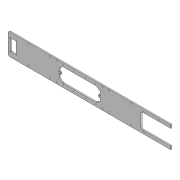
# Autodesk Inventor part: SlipersLåda 211018006
Saved by Autodesk Inventor 2020 (Build 240168000, 168)
## iProperties
Created: 2021-10-19
Part Number: SlipersLåda 211018006
Material: Generic
Document SubType Name: Modeling
Designer: dicpet001
Density: 1 g/cm^3
Appearance: Default
Author: dicpet001
Autodesk Inventor part; units mm, degrees
ref_plane "YZ Plane" through (0, 0, 0) normal (1, 0, 0) x (0, 1, 0)
ref_plane "XZ Plane" through (0, 0, 0) normal (0, 1, 0) x (-1, 0, 0)
ref_plane "XY Plane" through (0, 0, 0) normal (0, 0, 1) x (1, 0, 0)
sketch "Sketch1" plane through (0, 0, 0) normal (0, 0, 1) x (1, 0, 0)
  line L0 (0, 288.6985) -> (0, -288.6985) projected
  line L1 (-2107.4558, 0) -> (2101.2426, 0) projected
  line L2 (-1470, 200) -> (1500, 200)
  line L3 (1500, 200) -> (1500, -200)
  line L4 (1500, -200) -> (-1470, -200)
  line L5 (-1500, -170) -> (-1500, 170)
  arc A0 (-1470, 200) -> (-1500, 170) centre (-1470, 170) ccw
  arc A1 (-1500, -170) -> (-1470, -200) centre (-1470, -170) ccw
  line L6 (-1445, 110) -> (-1365, 110)
  line L7 (-1350, 95) -> (-1350, -95)
  line L8 (-1365, -110) -> (-1445, -110)
  line L9 (-1460, -95) -> (-1460, 95)
  arc A2 (-1445, 110) -> (-1460, 95) centre (-1445, 95) ccw
  arc A3 (-1350, 95) -> (-1365, 110) centre (-1365, 95) ccw
  arc A4 (-1365, -110) -> (-1350, -95) centre (-1365, -95) ccw
  arc A5 (-1460, -95) -> (-1445, -110) centre (-1445, -95) ccw
  point P0 (0, 0)
  point P1 (-1500, 200)
  point P2 (-1500, -200)
  point P3 (-1465, 115)
  point P4 (-1345, 115)
  point P5 (-1345, -115)
  point P6 (-1465, -115)
  dimension "d0" = 400
  dimension "d1" = 3000
  dimension "d2" = 30
  dimension "d3" = 110
  dimension "d4" = 220
  dimension "d5" = 15
  dimension "d8" = 230
  dimension "d9" = 120
  dimension "d10" = 5
  dimension "d11" = 5
  dimension "d12" = 40
  constraints: 16 end point, 12 point on circle, 12 tangent, 6 centre point, 4 equal radius, 4 parallel, 4 point on line, 2 horizontal, 2 horizontal alignment, 2 perpendicular, 2 vertical alignment, 3 other
  measures "d0" distance of point (-1500, -200) point (-1500, 200)
  measures "d1" distance of point (-1500, 200) L2.end
  measures "d2" radius of A0
  measures "d3" distance between parallel lines of L7 L9
  measures "d4" distance between parallel lines of L8 L6
  measures "d5" radius of A2
  measures "d8" distance of point (-1345, -115) point (-1345, 115)
  measures "d9" distance of point (-1465, -115) point (-1345, -115)
  measures "d10" distance from line of L8 point (-1465, -115)
  measures "d11" distance from line of L9 point (-1465, -115)
  measures "d12" distance between parallel lines of L9 L5
extrude "Extrusion1" add sketch "Sketch1" against normal blind 20 contours L2 L3 L1 L0 | L0 L1 L7 A3 L6 A2 L9 L5 A0 L2 | L1 L3 L4 L0 | L0 L4 A1 L5 L1 L9 A5 L8 A4 L7
hole "Hole1" at (-1465, 115, 0) at (-1345, 115, 0) at (-1345, -115, 0) at (-1465, -115, 0) direction (0, 0, -1) diameter 10.106 end through all thread size "M12x1.75" class "6H" standard "ISO Metric profile"
sketch "Sketch2" plane through (0, 0, 0) normal (0, 0, 1) x (1, 0, 0)
  circle A0 centre (-1345, -115) radius 5.053 projected
  circle A1 centre (-1465, 115) radius 5.053 projected
  circle A2 centre (-1345, 115) radius 5.053 projected
  circle A3 centre (-1465, -115) radius 5.053 projected
  line L0 (-1500, 170) -> (-1500, -170) projected
  arc A4 (-1500, -170) -> (-1470, -200) centre (-1470, -170) ccw projected
  line L1 (-1470, -200) -> (1500, -200) projected
  line L2 (1500, -200) -> (1500, 200) projected
  line L3 (1500, 200) -> (-1470, 200) projected
  arc A5 (-1470, 200) -> (-1500, 170) centre (-1470, 170) ccw projected
  arc A6 (-1460, -95) -> (-1445, -110) centre (-1445, -95) ccw projected
  line L4 (-1460, -95) -> (-1460, 95) projected
  arc A7 (-1445, 110) -> (-1460, 95) centre (-1445, 95) ccw projected
  line L5 (-1445, 110) -> (-1365, 110) projected
  arc A8 (-1350, 95) -> (-1365, 110) centre (-1365, 95) ccw projected
  line L6 (-1350, 95) -> (-1350, -95) projected
  arc A9 (-1365, -110) -> (-1350, -95) centre (-1365, -95) ccw projected
  line L7 (-1365, -110) -> (-1445, -110) projected
  line L8 (1500, 140) -> (975, 140)
  line L9 (950, 115) -> (950, -115)
  line L10 (975, -140) -> (1500, -140)
  line L11 (1500, -140) -> (1500, 140)
  line L12 (0, 288.6985) -> (0, -288.6985) projected
  line L13 (-2107.4558, 0) -> (2101.2426, 0) projected
  arc A10 (975, 140) -> (950, 115) centre (975, 115) ccw
  arc A11 (950, -115) -> (975, -140) centre (975, -115) ccw
  circle A12 centre (1270, 175) radius 3.5
  point P0 (0, 0)
  point P1 (998, 160)
  point P2 (1025, 160)
  point P3 (998, -160)
  point P4 (1025, -160)
  point P5 (1270, 160)
  dimension "d22" = 550
  dimension "d23" = 280
  dimension "d24" = 25
  dimension "d25" = 7
  dimension "d26" = 230
  dimension "d27" = 320
  dimension "d28" = 27
  dimension "d29" = 475
  dimension "d30" = 230
  dimension "d31" = 15
  constraints: 8 end point, 4 point on circle, 4 tangent, 3 centre point, 3 horizontal alignment, 2 parallel, 2 vertical alignment, 1 equal radius, 1 horizontal, 1 perpendicular, 1 point on line, 1 symmetric about line, 1 other
  measures "d22" distance between parallel lines of L2 L9
  measures "d23" distance between parallel lines of L10 L8
  measures "d24" radius of A10
  measures "d25" diameter of A12
  measures "d26" distance from line of L2 A12.centre
  measures "d27" distance of point (1025, -160) point (1025, 160)
  measures "d28" distance of point (998, 160) point (1025, 160)
  measures "d29" distance from line of L2 point (1025, -160)
  measures "d30" distance from line of L2 point (1270, 160)
  measures "d31" distance of A12.centre point (1270, 160)
extrude "Extrusion2" cut sketch "Sketch2" against normal blind 20 contours L2 L13 L9 A10 L8 | L13 L2 L10 A11 L9 | A12
hole "Hole2" at (998, 160, 0) at (1025, 160, 0) at (998, -160, 0) at (1025, -160, 0) at (1270, 160, 0) direction (0, 0, -1) diameter 10.106 end through all thread size "M12x1.75" class "6H" standard "ISO Metric profile"
sketch "Sketch3" plane through (0, 0, 0) normal (0, 0, 1) x (1, 0, 0)
  line L0 (0, 1076.2642) -> (0, -784.2642) projected
  line L1 (-2100, 0) -> (2100, 0) projected
  line L2 (1500, -200) -> (1500, -140) projected
  line L3 (-1470, -200) -> (1500, -200) projected
  arc A0 (-491.6194, -128.7689) -> (-483.7482, -131) centre (-483.7482, -116) ccw
  line L4 (-491.6194, 128.7689) -> (-553.8712, 90.3945)
  arc A1 (-483.7482, 131) -> (-491.6194, 128.7689) centre (-483.7482, 116) ccw
  line L5 (-483.7482, 131) -> (-183, 131)
  arc A2 (-531, 2.5) -> (-546, 17.5) centre (-546, 2.5) ccw
  line L6 (-561, 32.5) -> (-561, 77.6256)
  arc A3 (-546, -17.5) -> (-561, -32.5) centre (-546, -32.5) ccw
  arc A4 (-553.8712, 90.3945) -> (-561, 77.6256) centre (-546, 77.6256) ccw
  line L7 (-561, -77.6256) -> (-561, -32.5)
  line L8 (-491.6194, -128.7689) -> (-553.8712, -90.3945)
  line L9 (-546, 17.5) -> (-546, 17.5)
  arc A5 (-561, 32.5) -> (-546, 17.5) centre (-546, 32.5) ccw
  line L10 (-183, -131) -> (-483.7482, -131)
  line L11 (-531, 2.5) -> (-531, -2.5)
  line L12 (-546, -17.5) -> (-546, -17.5)
  arc A6 (-546, -17.5) -> (-531, -2.5) centre (-546, -2.5) ccw
  line L13 (180, -17.5) -> (180, -17.5)
  arc A7 (165, -2.5) -> (180, -17.5) centre (180, -2.5) ccw
  circle A8 centre (-546, 0) radius 4.5
  arc A9 (-561, -77.6256) -> (-553.8712, -90.3945) centre (-546, -77.6256) ccw
  line L14 (-183, -131) -> (117.7482, -131)
  line L15 (117.7482, 131) -> (-183, 131)
  arc A10 (117.7482, -131) -> (125.6194, -128.7689) centre (117.7482, -116) ccw
  arc A11 (125.6194, 128.7689) -> (117.7482, 131) centre (117.7482, 116) ccw
  line L16 (165, 2.5) -> (165, -2.5)
  line L17 (180, 17.5) -> (180, 17.5)
  arc A12 (180, 17.5) -> (165, 2.5) centre (180, 2.5) ccw
  circle A13 centre (180, 0) radius 4.5
  arc A14 (187.8712, -90.3945) -> (195, -77.6256) centre (180, -77.6256) ccw
  arc A15 (195, -32.5) -> (180, -17.5) centre (180, -32.5) ccw
  arc A16 (180, 17.5) -> (195, 32.5) centre (180, 32.5) ccw
  line L18 (125.6194, 128.7689) -> (187.8712, 90.3945)
  arc A17 (195, 77.6256) -> (187.8712, 90.3945) centre (180, 77.6256) ccw
  line L19 (195, -77.6256) -> (195, -32.5)
  line L20 (125.6194, -128.7689) -> (187.8712, -90.3945)
  line L21 (195, 32.5) -> (195, 77.6256)
  line L22 (-183, 131) -> (-183, -131)
  point P0 (-620.9638, -518.4744)
  point P1 (-488, 131)
  point P2 (-561, 86)
  point P3 (-488, -131)
  point P4 (-561, -86)
  point P5 (122, 131)
  point P6 (195, -86)
  point P7 (195, 86)
  point P8 (122, -131)
  point P9 (200, -16)
  point P10 (200, 16)
  point P11 (-566, -16)
  point P12 (-566, 16)
  point P13 (-293, 810.4744)
  point P14 (-482, 810.4744)
  point P15 (-293, 161)
  point P16 (-482, 161)
  point P17 (-293, -161)
  point P18 (-482, -161)
  point P19 (-73, 161)
  point P20 (116, 161)
  point P21 (116, -161)
  point P22 (-73, -161)
  dimension "d76" = 262
  dimension "d77" = 35
  dimension "d78" = 15
  dimension "d79" = 32
  dimension "d80" = 189
  dimension "d81" = 9
  dimension "d82" = 20
  dimension "d83" = 1305
  dimension "d86" = 756
  dimension "d87" = 195
  dimension "d88" = 183
  dimension "d89" = 110
  dimension "d90" = 189
  dimension "d91" = 161
  constraints: 38 end point, 32 point on circle, 18 centre point, 16 point on line, 16 tangent, 7 equal radius, 6 symmetric about line, 2 horizontal, 2 horizontal alignment, 2 perpendicular, 2 vertical, 1 parallel
  measures "d76" distance between parallel lines of L5 L10
  measures "d77" distance between parallel lines of L12 L9
  measures "d78" radius of A0
  measures "d79" distance of point (-566, 16) point (-566, -16)
  measures "d80" distance of point (-482, 810.474) point (-293, 810.474)
  measures "d81" diameter of A8
  measures "d82" horizontal distance of A8.centre point (-566, 16)
  measures "d83" distance between parallel lines of L2 L19
  measures "d86" distance between parallel lines of L21 L6
  measures "d87" distance between parallel lines of L21 L0
  measures "d88" distance between parallel lines of L0 L22
  measures "d89" distance from line of L22 point (-293, 161)
  measures "d90" distance of point (-482, 161) point (-293, 161)
  measures "d91" distance from line of point (-482, 161) L1
extrude "Extrusion3" cut sketch "Sketch3" against normal blind 20
hole "Hole4" at (-482, 810.4744, 0) at (-293, 810.4744, 0) at (-566, 16, 0) at (-566, -16, 0) at (200, 16, 0) at (200, -16, 0) at (-293, 161, 0) at (-482, 161, 0) at (-482, -161, 0) at (-293, -161, 0) at (116, 161, 0) at (-73, 161, 0) at (116, -161, 0) at (-73, -161, 0) direction (0, 0, -1) diameter 10.106 end through all thread size "M12x1.75" class "6H" standard "ISO Metric profile"
sketch "Sketch4" plane through (0, 0, 0) normal (0, 0, 1) x (1, 0, 0)
  circle A0 centre (116, -161) radius 5.053 projected
  circle A1 centre (116, 161) radius 5.053 projected
  circle A2 centre (-482, -161) radius 5.053 projected
  circle A3 centre (-293, 161) radius 5.053 projected
  circle A4 centre (200, 16) radius 5.053 projected
  circle A5 centre (-566, 16) radius 5.053 projected
  circle A6 centre (-566, -16) radius 5.053 projected
  circle A7 centre (200, -16) radius 5.053 projected
  circle A8 centre (-482, 161) radius 5.053 projected
  circle A9 centre (-293, -161) radius 5.053 projected
  circle A10 centre (-73, 161) radius 5.053 projected
  circle A11 centre (-73, -161) radius 5.053 projected
  circle A12 centre (180, 0) radius 4.5 projected
  circle A13 centre (-546, 0) radius 4.5 projected
  arc A14 (-553.8712, 90.3945) -> (-561, 77.6256) centre (-546, 77.6256) ccw projected
  line L0 (-553.8712, 90.3945) -> (-491.6194, 128.7689) projected
  arc A15 (-483.7482, 131) -> (-491.6194, 128.7689) centre (-483.7482, 116) ccw projected
  line L1 (-483.7482, 131) -> (117.7482, 131) projected
  arc A16 (125.6194, 128.7689) -> (117.7482, 131) centre (117.7482, 116) ccw projected
  line L2 (125.6194, 128.7689) -> (187.8712, 90.3945) projected
  arc A17 (195, 77.6256) -> (187.8712, 90.3945) centre (180, 77.6256) ccw projected
  line L3 (195, 77.6256) -> (195, 32.5) projected
  arc A18 (180, 17.5) -> (195, 32.5) centre (180, 32.5) ccw projected
  arc A19 (180, 17.5) -> (165, 2.5) centre (180, 2.5) ccw projected
  line L4 (165, 2.5) -> (165, -2.5) projected
  arc A20 (165, -2.5) -> (180, -17.5) centre (180, -2.5) ccw projected
  arc A21 (195, -32.5) -> (180, -17.5) centre (180, -32.5) ccw projected
  line L5 (195, -32.5) -> (195, -77.6256) projected
  arc A22 (187.8712, -90.3945) -> (195, -77.6256) centre (180, -77.6256) ccw projected
  line L6 (187.8712, -90.3945) -> (125.6194, -128.7689) projected
  arc A23 (117.7482, -131) -> (125.6194, -128.7689) centre (117.7482, -116) ccw projected
  line L7 (117.7482, -131) -> (-483.7482, -131) projected
  arc A24 (-491.6194, -128.7689) -> (-483.7482, -131) centre (-483.7482, -116) ccw projected
  line L8 (-491.6194, -128.7689) -> (-553.8712, -90.3945) projected
  arc A25 (-561, -77.6256) -> (-553.8712, -90.3945) centre (-546, -77.6256) ccw projected
  line L9 (-561, -77.6256) -> (-561, -32.5) projected
  arc A26 (-546, -17.5) -> (-561, -32.5) centre (-546, -32.5) ccw projected
  arc A27 (-546, -17.5) -> (-531, -2.5) centre (-546, -2.5) ccw projected
  line L10 (-531, -2.5) -> (-531, 2.5) projected
  arc A28 (-531, 2.5) -> (-546, 17.5) centre (-546, 2.5) ccw projected
  arc A29 (-561, 32.5) -> (-546, 17.5) centre (-546, 32.5) ccw projected
  line L11 (-561, 32.5) -> (-561, 77.6256) projected
  circle A30 centre (1025, -160) radius 5.053 projected
  circle A31 centre (1025, 160) radius 5.053 projected
  circle A32 centre (998, 160) radius 5.053 projected
  circle A33 centre (998, -160) radius 5.053 projected
  circle A34 centre (1270, 160) radius 5.053 projected
  line L12 (975, 140) -> (1500, 140) projected
  line L13 (1500, 140) -> (1500, 200) projected
  line L14 (1500, 200) -> (-1470, 200) projected
  arc A35 (-1470, 200) -> (-1500, 170) centre (-1470, 170) ccw projected
  line L15 (-1500, 170) -> (-1500, -170) projected
  arc A36 (-1500, -170) -> (-1470, -200) centre (-1470, -170) ccw projected
  line L16 (-1470, -200) -> (1500, -200) projected
  line L17 (1500, -200) -> (1500, -140) projected
  line L18 (1500, -140) -> (975, -140) projected
  arc A37 (950, -115) -> (975, -140) centre (975, -115) ccw projected
  line L19 (950, -115) -> (950, 115) projected
  arc A38 (975, 140) -> (950, 115) centre (975, 115) ccw projected
  circle A39 centre (1270, 175) radius 3.5 projected
  circle A40 centre (-1345, -115) radius 5.053 projected
  circle A41 centre (-1465, 115) radius 5.053 projected
  circle A42 centre (-1345, 115) radius 5.053 projected
  circle A43 centre (-1465, -115) radius 5.053 projected
  arc A44 (-1460, -95) -> (-1445, -110) centre (-1445, -95) ccw projected
  line L20 (-1460, -95) -> (-1460, 95) projected
  arc A45 (-1445, 110) -> (-1460, 95) centre (-1445, 95) ccw projected
  line L21 (-1445, 110) -> (-1365, 110) projected
  arc A46 (-1350, 95) -> (-1365, 110) centre (-1365, 95) ccw projected
  line L22 (-1350, 95) -> (-1350, -95) projected
  arc A47 (-1365, -110) -> (-1350, -95) centre (-1365, -95) ccw projected
  line L23 (-1365, -110) -> (-1445, -110) projected
  line L24 (117.7482, 131) -> (-483.7482, 131) projected
  line L25 (-183, 131) -> (-183, -131)
  line L26 (0, 288.6985) -> (0, -288.6985) projected
  line L27 (-2107.4558, 0) -> (2101.2426, 0) projected
  point P0 (0, 0)
  point P1 (-603, 175)
  point P2 (-728, 175)
  point P3 (-1128, 175)
  point P4 (-603, -175)
  point P5 (-728, -175)
  point P6 (-1128, -175)
  point P7 (237, 175)
  point P8 (362, 175)
  point P9 (762, 175)
  point P10 (762, -175)
  point P11 (362, -175)
  point P12 (237, -175)
  dimension "d99" = 420
  dimension "d100" = 545
  dimension "d101" = 400
  dimension "d109" = 175
  constraints: 9 symmetric about line, 2 end point, 2 horizontal alignment, 2 midpoint
  measures "d99" distance from line of point (-603, 175) L25
  measures "d100" distance from line of point (-728, 175) L25
  measures "d101" distance of point (-1128, 175) point (-728, 175)
  measures "d109" distance from line of point (-603, 175) L27
hole "Hole5" at (-603, 175, 0) at (-728, 175, 0) at (-1128, 175, 0) at (-1128, -175, 0) at (-728, -175, 0) at (-603, -175, 0) at (237, -175, 0) at (362, -175, 0) at (762, -175, 0) at (762, 175, 0) at (362, 175, 0) at (237, 175, 0) direction (0, 0, -1) diameter 30 end through all
sketch "Sketch5" plane through (0, 0, 0) normal (0, 0, 1) x (1, 0, 0)
  circle A0 centre (362, 175) radius 15 projected
  circle A1 centre (762, -175) radius 15 projected
  circle A2 centre (237, -175) radius 15 projected
  circle A3 centre (-728, -175) radius 15 projected
  circle A4 centre (-1128, 175) radius 15 projected
  circle A5 centre (-603, 175) radius 15 projected
  circle A6 centre (-728, 175) radius 15 projected
  circle A7 centre (-1128, -175) radius 15 projected
  circle A8 centre (-603, -175) radius 15 projected
  circle A9 centre (362, -175) radius 15 projected
  circle A10 centre (762, 175) radius 15 projected
  circle A11 centre (237, 175) radius 15 projected
  circle A12 centre (116, -161) radius 5.053 projected
  circle A13 centre (116, 161) radius 5.053 projected
  circle A14 centre (-482, -161) radius 5.053 projected
  circle A15 centre (-293, 161) radius 5.053 projected
  circle A16 centre (200, 16) radius 5.053 projected
  circle A17 centre (-566, 16) radius 5.053 projected
  circle A18 centre (-566, -16) radius 5.053 projected
  circle A19 centre (200, -16) radius 5.053 projected
  circle A20 centre (-482, 161) radius 5.053 projected
  circle A21 centre (-293, -161) radius 5.053 projected
  circle A22 centre (-73, 161) radius 5.053 projected
  circle A23 centre (-73, -161) radius 5.053 projected
  circle A24 centre (180, 0) radius 4.5 projected
  circle A25 centre (-546, 0) radius 4.5 projected
  arc A26 (-553.8712, 90.3945) -> (-561, 77.6256) centre (-546, 77.6256) ccw projected
  line L0 (-553.8712, 90.3945) -> (-491.6194, 128.7689) projected
  arc A27 (-483.7482, 131) -> (-491.6194, 128.7689) centre (-483.7482, 116) ccw projected
  line L1 (-483.7482, 131) -> (117.7482, 131) projected
  arc A28 (125.6194, 128.7689) -> (117.7482, 131) centre (117.7482, 116) ccw projected
  line L2 (125.6194, 128.7689) -> (187.8712, 90.3945) projected
  arc A29 (195, 77.6256) -> (187.8712, 90.3945) centre (180, 77.6256) ccw projected
  line L3 (195, 77.6256) -> (195, 32.5) projected
  arc A30 (180, 17.5) -> (195, 32.5) centre (180, 32.5) ccw projected
  arc A31 (180, 17.5) -> (165, 2.5) centre (180, 2.5) ccw projected
  line L4 (165, 2.5) -> (165, -2.5) projected
  arc A32 (165, -2.5) -> (180, -17.5) centre (180, -2.5) ccw projected
  arc A33 (195, -32.5) -> (180, -17.5) centre (180, -32.5) ccw projected
  line L5 (195, -32.5) -> (195, -77.6256) projected
  arc A34 (187.8712, -90.3945) -> (195, -77.6256) centre (180, -77.6256) ccw projected
  line L6 (187.8712, -90.3945) -> (125.6194, -128.7689) projected
  arc A35 (117.7482, -131) -> (125.6194, -128.7689) centre (117.7482, -116) ccw projected
  line L7 (117.7482, -131) -> (-483.7482, -131) projected
  arc A36 (-491.6194, -128.7689) -> (-483.7482, -131) centre (-483.7482, -116) ccw projected
  line L8 (-491.6194, -128.7689) -> (-553.8712, -90.3945) projected
  arc A37 (-561, -77.6256) -> (-553.8712, -90.3945) centre (-546, -77.6256) ccw projected
  line L9 (-561, -77.6256) -> (-561, -32.5) projected
  arc A38 (-546, -17.5) -> (-561, -32.5) centre (-546, -32.5) ccw projected
  arc A39 (-546, -17.5) -> (-531, -2.5) centre (-546, -2.5) ccw projected
  line L10 (-531, -2.5) -> (-531, 2.5) projected
  arc A40 (-531, 2.5) -> (-546, 17.5) centre (-546, 2.5) ccw projected
  arc A41 (-561, 32.5) -> (-546, 17.5) centre (-546, 32.5) ccw projected
  line L11 (-561, 32.5) -> (-561, 77.6256) projected
  circle A42 centre (1025, -160) radius 5.053 projected
  circle A43 centre (1025, 160) radius 5.053 projected
  circle A44 centre (998, 160) radius 5.053 projected
  circle A45 centre (998, -160) radius 5.053 projected
  circle A46 centre (1270, 160) radius 5.053 projected
  line L12 (975, 140) -> (1500, 140) projected
  line L13 (1500, 140) -> (1500, 200) projected
  line L14 (1500, 200) -> (-1470, 200) projected
  arc A47 (-1470, 200) -> (-1500, 170) centre (-1470, 170) ccw projected
  line L15 (-1500, 170) -> (-1500, -170) projected
  arc A48 (-1500, -170) -> (-1470, -200) centre (-1470, -170) ccw projected
  line L16 (-1470, -200) -> (1500, -200) projected
  line L17 (1500, -200) -> (1500, -140) projected
  line L18 (1500, -140) -> (975, -140) projected
  arc A49 (950, -115) -> (975, -140) centre (975, -115) ccw projected
  line L19 (950, -115) -> (950, 115) projected
  arc A50 (975, 140) -> (950, 115) centre (975, 115) ccw projected
  circle A51 centre (1270, 175) radius 3.5 projected
  circle A52 centre (-1345, -115) radius 5.053 projected
  circle A53 centre (-1465, 115) radius 5.053 projected
  circle A54 centre (-1345, 115) radius 5.053 projected
  circle A55 centre (-1465, -115) radius 5.053 projected
  arc A56 (-1460, -95) -> (-1445, -110) centre (-1445, -95) ccw projected
  line L20 (-1460, -95) -> (-1460, 95) projected
  arc A57 (-1445, 110) -> (-1460, 95) centre (-1445, 95) ccw projected
  line L21 (-1445, 110) -> (-1365, 110) projected
  arc A58 (-1350, 95) -> (-1365, 110) centre (-1365, 95) ccw projected
  line L22 (-1350, 95) -> (-1350, -95) projected
  arc A59 (-1365, -110) -> (-1350, -95) centre (-1365, -95) ccw projected
  line L23 (-1365, -110) -> (-1445, -110) projected
  arc A60 (-561, 32.5) -> (-546, 17.5) centre (-546, 32.5) ccw
  arc A61 (-531, 2.5) -> (-546, 17.5) centre (-546, 2.5) ccw
  line L24 (-531, 2.5) -> (-531, -2.5) projected
  line L25 (-531, 2.5) -> (-531, 0)
  line L26 (-531, 0) -> (-511.8898, 0)
  line L27 (-483.7482, 131) -> (117.7482, 131) projected
  arc A62 (-561, 40) -> (-546, 25) centre (-546, 40) ccw
  arc A63 (-531, 10) -> (-546, 25) centre (-546, 10) ccw
  line L28 (-531, 10) -> (-531, 2.5)
  line L29 (-561, 32.5) -> (-561, 40)
  line L30 (-561, 32.5) -> (-561, 77.6256) projected
  line L31 (-531, 2.5) -> (-531, -2.5)
  arc A64 (-546, -17.5) -> (-531, -2.5) centre (-546, -2.5) ccw
  arc A65 (-546, -17.5) -> (-561, -32.5) centre (-546, -32.5) ccw
  line L32 (-531, -2.5) -> (-531, 2.5)
  line L33 (-531, -2.5) -> (-531, 0)
  arc A66 (-546, -25) -> (-561, -40) centre (-546, -40) ccw
  arc A67 (-546, -25) -> (-531, -10) centre (-546, -10) ccw
  line L34 (-531, -10) -> (-531, -2.5)
  line L35 (-561, -32.5) -> (-561, -40)
  line L36 (165, 2.5) -> (165, -2.5) projected
  arc A68 (180, 17.5) -> (195, 32.5) centre (180, 32.5) ccw
  line L37 (165, 2.5) -> (165, 10)
  arc A69 (180, 25) -> (165, 10) centre (180, 10) ccw
  arc A70 (180, 25) -> (195, 40) centre (180, 40) ccw
  line L38 (195, 77.6256) -> (195, 32.5) projected
  line L39 (195, 40) -> (195, 32.5)
  arc A71 (195, -32.5) -> (180, -17.5) centre (180, -32.5) ccw
  arc A72 (195, -32.5) -> (180, -17.5) centre (180, -32.5) ccw
  line L40 (165, -2.5) -> (165, -10)
  arc A73 (165, -10) -> (180, -25) centre (180, -10) ccw
  arc A74 (195, -40) -> (180, -25) centre (180, -40) ccw
  line L41 (195, -40) -> (195, -32.5)
  arc A75 (180, 17.5) -> (165, 2.5) centre (180, 2.5) ccw
  arc A76 (165, -2.5) -> (180, -17.5) centre (180, -2.5) ccw
  point P0 (0, 0)
  point P1 (-531, -2.5)
  point P2 (200, -16)
  point P3 (165, 2.5)
  constraints: 37 point on circle, 26 end point, 17 centre point, 10 symmetric about line, 7 tangent, 3 concentric, 2 coincident, 2 collinear, 1 horizontal, 1 midpoint, 4 other
extrude "Extrusion4" add sketch "Sketch5" against normal blind 20 contours A62 A63 L28 A40 A41 L11 | L34 A67 A66 L9 A38 A39 | L3 A30 A31 L37 A69 A70 | A32 A33 L5 A74 A73 L40
body "Solid1"
